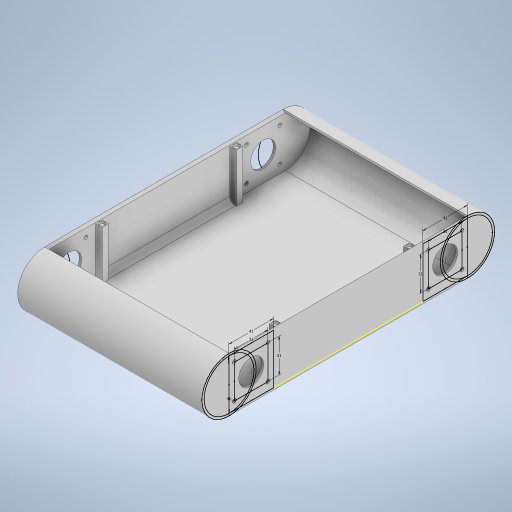
# Autodesk Inventor part: bottom
Saved by Autodesk Inventor 2024 (Build 280153020, 153B)
## iProperties
Created: 2025-07-09
Part Number: bottom
Material: Generic
Document SubType Name: Modeling
Designer: andre
Density: 1 g/cm^3
Appearance: Default
Author: andre
Autodesk Inventor part; units mm, degrees
ref_plane "YZ Plane" through (0, 0, 0) normal (1, 0, 0) x (0, 1, 0)
ref_plane "XZ Plane" through (0, 0, 0) normal (0, 1, 0) x (-1, 0, 0)
ref_plane "XY Plane" through (0, 0, 0) normal (0, 0, 1) x (1, 0, 0)
sketch "Sketch1" plane through (0, 0, 0) normal (0, 1, 0) x (-1, 0, 0)
  line L0 (0, 0) -> (170, 0)
  line L1 (170, 0) -> (170, -220)
  line L2 (170, -220) -> (0, -220)
  line L3 (0, -220) -> (0, 0)
  dimension "d0" = 170
  dimension "d1" = 220
  constraints: 8 end point, 2 parallel, 1 horizontal, 1 perpendicular
  measures "d0" distance of L1.end L2.end
  measures "d1" distance of L0.end L1.end
extrude "base" add sketch "Sketch1" along normal blind 2
sketch "Sketch2" plane through (0, 2, 0) normal (0, 1, 0) x (1, 0, 0)
  line L0 (0, 0) -> (0, 220) projected
  line L1 (0, 220) -> (-170, 220) projected
  line L2 (0, 0) -> (-2, 0)
  line L3 (-2, 0) -> (-2, 220)
  line L4 (-2, 220) -> (0, 220)
  line L5 (0, 220) -> (0, 0)
  line L6 (-170, 220) -> (-170, 0) projected
  line L7 (-170, 0) -> (-168, 0)
  line L8 (-168, 0) -> (-168, 220)
  line L9 (-168, 220) -> (-170, 220)
  line L10 (-170, 220) -> (-170, 0)
  dimension "d4" = 2
  dimension "d5" = 2
  constraints: 16 end point, 4 parallel, 2 horizontal, 2 perpendicular, 2 point on line
  measures "d4" distance of L3.end L4.end
  measures "d5" distance of L9.end L8.end
extrude "walls" add sketch "Sketch2" along normal blind 48
sketch "rounded_wall" plane through (0, 0, 0) normal (1, 0, 0) x (0, 0, -1)
  line L0 (0, 0) -> (0, 50) projected
  line L1 (0, 0) -> (0, 50)
  circle A0 centre (0, 25) radius 25
  circle A1 centre (0, 25) radius 23
  line L2 (220, 0) -> (220, 50) projected
  line L3 (220, 0) -> (220, 50)
  circle A2 centre (220, 25) radius 25
  line L4 (220, 2) -> (220, 50) projected
  circle A3 centre (220, 25) radius 23
  point P0 (0, 2)
  point P1 (0, 48)
  point P2 (220, 48)
  dimension "d8" = 46
  constraints: 4 end point, 2 coincident, 2 midpoint, 1 centre point, 1 collinear, 1 vertical, 9 other
  measures "d8" diameter of A1
extrude "rounded_wall_extrusion" add sketch "rounded_wall" against normal blind 170 contours A0 L0 A1 | L2 A3 A2 picked at (-24.1559, 25.9241) picked at (243.9322, 21.4397)
extrude "rounded_wall_side1_extrusion" add sketch "rounded_wall" against normal blind 2 contours A1 L0 | L2 A3 picked at (-13.0084, 23.4205) picked at (235.581, 24.2074)
sketch "rounded_wall_side2" plane through (-170, 0, -220) normal (-1, 0, 0) x (0, 0, 1)
  line L0 (220, 2) -> (220, 48) projected
  line L1 (220, 48) -> (220, 2)
  arc A0 (220, 2) -> (220, 48) centre (220, 25) ccw projected
  circle A1 centre (220, 25) radius 23
  line L2 (0, 0) -> (220, 0) projected
  line L3 (0, 48) -> (0, 2)
  line L4 (0, 48) -> (0, 2)
  arc A2 (0, 48) -> (0, 2) centre (0, 25) ccw projected
  circle A3 centre (0, 25) radius 23
  point P0 (220, 4.5)
  constraints: 6 end point, 2 midpoint, 2 vertical alignment, 1 collinear, 1 perpendicular, 1 vertical, 4 other
extrude "rounded_wall_side2_extrusion" add sketch "rounded_wall_side2" against normal blind 2 contours L0 A0 | L3 A2
sketch "holes" plane through (0, 25, -220) normal (1, 0, 0) x (0, 0, -1)
  arc A0 (-220, 23) -> (-220, -23) centre (-220, 0) ccw projected
  line L0 (-220, -23) -> (-179, -23)
  line L1 (-179, -23) -> (-179, 23)
  line L2 (-179, 23) -> (-220, 23)
  line L3 (-220, 23) -> (-220, -23)
  line L4 (-220, -23) -> (0, -23) projected
  line L5 (0, -23) -> (-41, -23)
  line L6 (-41, -23) -> (-41, 23)
  line L7 (-41, 23) -> (0, 23)
  line L8 (0, 23) -> (0, -23)
  line L9 (-5, -15.5) -> (-36, -15.5)
  line L10 (-36, -15.5) -> (-36, 15.5)
  line L11 (-36, 15.5) -> (-5, 15.5)
  line L12 (-5, 15.5) -> (-5, -15.5)
  arc A1 (0, -23) -> (0, 23) centre (0, 0) ccw projected
  line L13 (-215, -15.5) -> (-184, -15.5)
  line L14 (-184, -15.5) -> (-184, 15.5)
  line L15 (-184, 15.5) -> (-215, 15.5)
  line L16 (-215, 15.5) -> (-215, -15.5)
  arc A2 (-220, 25) -> (-220, -25) centre (-220, 0) ccw projected
  point P0 (-20.5, -15.5)
  point P1 (-20.5, -23)
  point P2 (-5, 0)
  point P3 (23, 0)
  point P4 (-215, 0)
  point P5 (-245, 0)
  point P6 (-199.5, -15.5)
  point P7 (-199.5, -23)
  point P8 (-199.5, 0)
  point P9 (-20.5, 0)
  point P10 (-199.5, 23)
  dimension "d15" = 41
  dimension "d16" = 41
  dimension "d17" = 31
  dimension "d18" = 31
  dimension "d19" = 31
  dimension "d20" = 31
  constraints: 32 end point, 8 coincident, 8 parallel, 7 midpoint, 4 horizontal, 4 perpendicular, 3 horizontal alignment, 2 point on circle, 2 vertical alignment
  measures "d15" distance of L2.end L1.end
  measures "d16" distance of L6.end L7.end
  measures "d17" distance of L10.end L11.end
  measures "d18" distance of L9.end L10.end
  measures "d19" distance of L15.end L14.end
  measures "d20" distance of L14.end L13.end
hole "shaft_holes" at (0, 25, -20.5) at (0, 25, -199.5) direction (-1, 0, 0) diameter 23 end through all
hole "motor_holes" at (0, 40.5, -5) at (0, 40.5, -36) at (0, 9.5, -5) at (0, 9.5, -36) at (0, 40.5, -184) at (0, 40.5, -215) at (0, 9.5, -215) at (0, 9.5, -184) direction (-1, 0, 0) diameter 3.5 end through all
sketch "Sketch7" plane through (0, 2, 0) normal (0, 1, 0) x (1, 0, 0)
  line L0 (-168, 220) -> (-168, 0) projected
  line L1 (-2, 220) -> (-2, 0) projected
  line L2 (-168, 45) -> (-2, 45)
  line L3 (-2, 45) -> (-2, 175)
  line L4 (-2, 175) -> (-168, 175)
  line L5 (-168, 175) -> (-168, 45)
  line L6 (-168, 175) -> (-162, 175)
  line L7 (-162, 175) -> (-162, 169)
  line L8 (-162, 169) -> (-168, 169)
  line L9 (-168, 169) -> (-168, 175)
  line L10 (-168, 45) -> (-162, 45)
  line L11 (-162, 45) -> (-162, 51)
  line L12 (-162, 51) -> (-168, 51)
  line L13 (-168, 51) -> (-168, 45)
  line L14 (-2, 175) -> (-8, 175)
  line L15 (-8, 175) -> (-8, 169)
  line L16 (-8, 169) -> (-2, 169)
  line L17 (-2, 169) -> (-2, 175)
  line L18 (-2, 45) -> (-8, 45)
  line L19 (-8, 45) -> (-8, 51)
  line L20 (-8, 51) -> (-2, 51)
  line L21 (-2, 51) -> (-2, 45)
  point P0 (0, 0)
  point P1 (-168, 110)
  point P2 (-2, 110)
  point P3 (-168, 169)
  point P4 (-162, 175)
  point P5 (-2, 51)
  point P6 (-2, 169)
  dimension "d35" = 130
  dimension "d36" = 6
  dimension "d37" = 6
  dimension "d38" = 6
  dimension "d39" = 6
  dimension "d40" = 6
  dimension "d41" = 6
  constraints: 40 end point, 10 parallel, 5 horizontal, 5 perpendicular, 4 point on line, 2 midpoint, 1 horizontal alignment
  measures "d35" distance of L3.end L2.end
  measures "d36" distance of L7.end L8.end
  measures "d37" distance of L6.end L7.end
  measures "d38" distance of L12.end L11.end
  measures "d39" distance of L11.end L10.end
  measures "d40" distance of L16.end L15.end
  measures "d41" distance of L15.end L14.end
extrude "columns" add sketch "Sketch7" along normal blind 45 contours L4 L7 L8 L0 | L12 L11 L2 L0 | L4 L1 L16 L15 | L19 L20 L1 L2
sketch "Sketch9" plane through (0, 47, 0) normal (0, 1, 0) x (1, 0, 0)
  line L0 (-8, 175) -> (-2, 175) projected
  line L1 (-8, 169) -> (-2, 169) projected
  line L2 (-8, 175) -> (-2, 175)
  line L3 (-2, 175) -> (-2, 169)
  line L4 (-2, 169) -> (-8, 169)
  line L5 (-8, 169) -> (-8, 175)
  line L6 (-8, 51) -> (-2, 51) projected
  line L7 (-2, 45) -> (-8, 45) projected
  line L8 (-2, 51) -> (-8, 51)
  line L9 (-8, 51) -> (-8, 45)
  line L10 (-8, 45) -> (-2, 45)
  line L11 (-2, 45) -> (-2, 51)
  line L12 (-162, 51) -> (-162, 45) projected
  line L13 (-168, 0) -> (-168, 220) projected
  line L14 (-162, 51) -> (-168, 51)
  line L15 (-168, 51) -> (-168, 45)
  line L16 (-168, 45) -> (-162, 45)
  line L17 (-162, 45) -> (-162, 51)
  line L18 (-162, 175) -> (-168, 175)
  line L19 (-168, 175) -> (-168, 169)
  line L20 (-168, 169) -> (-162, 169)
  line L21 (-162, 169) -> (-162, 175)
  point P0 (0, 0)
  point P1 (-165, 172)
  point P2 (-5, 172)
  point P3 (-5, 48)
  point P4 (-165, 48)
  constraints: 32 end point, 8 parallel, 6 point on line, 4 horizontal, 4 perpendicular
hole "magnet_holders" at (-165, 47, -172) at (-5, 47, -172) at (-5, 47, -48) at (-165, 47, -48) direction (0, -1, 0) diameter 5.5 depth 2
chamfer "chamfers" distance 2 angle 45 2 edges at (-2, 50, -110) (-168, 50, -110)
fillet "fillets" radius 5 2 edges at (-168, 2, -110) (-2, 2, -110)
body "Solid1"
